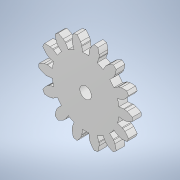
# Autodesk Inventor part: ｍ2歯数14ギアd3.99
Saved by Autodesk Inventor 2020.2 (Build 242310000, 310)
## iProperties
Created: 2020-03-09
Part Number: ｍ2歯数14ギアd3.99
Material: アルミニウム 2014-T4
Document SubType Name: Modeling
Designer: aoyam
Density: 2.8 g/cm^3
Appearance: サテン
Author: aoyam
Autodesk Inventor part; units mm, degrees
ref_plane "YZ Plane" through (0, 0, 0) normal (1, 0, 0) x (0, 1, 0)
ref_plane "XZ Plane" through (0, 0, 0) normal (0, 1, 0) x (-1, 0, 0)
ref_plane "XY Plane" through (0, 0, 0) normal (0, 0, 1) x (1, 0, 0)
sketch "スケッチ1" plane through (0, 0, 0) normal (0, 0, 1) x (1, 0, 0)
  arc A0 (3.0273, 14.808) -> (2.9636, 14.5404) centre (4.4576, 14.3261) ccw
  arc A1 (3.4088, 15.6481) -> (3.0273, 14.808) centre (7.0051, 13.5085) ccw
  arc A2 (4.6135, 17.1768) -> (3.4088, 15.6481) centre (9.7453, 11.8935) ccw
  arc A3 (0.4077, 14.5404) -> (0.344, 14.808) centre (-1.0864, 14.3261) ccw
  arc A4 (0.344, 14.808) -> (-0.0375, 15.6481) centre (-3.6338, 13.5085) ccw
  arc A5 (-0.0375, 15.6481) -> (-1.2422, 17.1768) centre (-6.374, 11.8935) ccw
  arc A6 (2.8028, 12.8925) -> (0.5685, 12.8925) centre (1.6856, 1.4469) ccw
  arc A7 (-1.2422, 17.1768) -> (-2.5014, 16.8894) centre (1.6856, 1.4469) ccw
  line L0 (2.8028, 12.8925) -> (2.9636, 14.5404)
  line L1 (0.5685, 12.8925) -> (0.4077, 14.5404)
  arc A8 (-6.0285, 13.4941) -> (-7.7772, 14.3487) centre (-10.1084, 7.362) ccw
  arc A9 (-7.7772, 14.3487) -> (-8.787, 13.5434) centre (1.6856, 1.4469) ccw
  arc A10 (-5.3203, 12.9027) -> (-6.0285, 13.4941) centre (-8.3404, 10.006) ccw
  arc A11 (-5.1468, 12.6893) -> (-5.3203, 12.9027) centre (-6.3999, 11.8479) ccw
  line L2 (-4.2869, 11.2744) -> (-5.1468, 12.6893)
  arc A12 (-2.9027, 14.067) -> (-2.844, 13.7982) centre (-1.405, 14.2534) ccw
  arc A13 (-2.9235, 14.9894) -> (-2.9027, 14.067) centre (1.2449, 14.6221) ccw
  arc A14 (-2.5014, 16.8894) -> (-2.9235, 14.9894) centre (4.4145, 14.3559) ccw
  line L3 (-2.2739, 12.2438) -> (-2.844, 13.7982)
  arc A15 (-2.2739, 12.2438) -> (-4.2869, 11.2744) centre (1.6856, 1.4469) ccw
  arc A16 (-10.4917, 8.954) -> (-12.4379, 8.9653) centre (-11.5069, 1.659) ccw
  arc A17 (-12.4379, 8.9653) -> (-12.9983, 7.8016) centre (1.6856, 1.4469) ccw
  arc A18 (-9.597, 8.7285) -> (-10.4917, 8.954) centre (-11.0611, 4.8083) ccw
  arc A19 (-9.3481, 8.6114) -> (-9.597, 8.7285) centre (-10.112, 7.3097) ccw
  line L4 (-7.9594, 7.7097) -> (-9.3481, 8.6114)
  arc A20 (-7.9239, 10.8264) -> (-7.7545, 10.6097) centre (-6.6554, 11.6442) ccw
  arc A21 (-8.343, 11.6485) -> (-7.9239, 10.8264) centre (-4.4279, 13.1261) ccw
  arc A22 (-8.787, 13.5434) -> (-8.343, 11.6485) centre (-1.4567, 14.2615) ccw
  line L5 (-6.5664, 9.4566) -> (-7.7545, 10.6097)
  arc A23 (-6.5664, 9.4566) -> (-7.9594, 7.7097) centre (1.6856, 1.4469) ccw
  arc A24 (-12.543, 2.927) -> (-14.3013, 2.0927) centre (-10.2925, -4.086) ccw
  arc A25 (-14.3013, 2.0927) -> (-14.3013, 0.8011) centre (1.6856, 1.4469) ccw
  arc A26 (-11.639, 3.112) -> (-12.543, 2.927) centre (-11.2573, -1.0552) ccw
  arc A27 (-11.3639, 3.1146) -> (-11.639, 3.112) centre (-11.4875, 1.6103) ccw
  line L6 (-9.7216, 2.9047) -> (-11.3639, 3.1146)
  arc A28 (-11.0419, 5.7281) -> (-10.7952, 5.6064) centre (-10.2538, 7.0153) ccw
  arc A29 (-11.7761, 6.2869) -> (-11.0419, 5.7281) centre (-8.8899, 9.317) ccw
  arc A30 (-12.9983, 7.8016) -> (-11.7761, 6.2869) centre (-6.7056, 11.6291) ccw
  line L7 (-9.2244, 5.0829) -> (-10.7952, 5.6064)
  arc A31 (-9.2244, 5.0829) -> (-9.7216, 2.9047) centre (1.6856, 1.4469) ccw
  arc A32 (-11.7761, -3.3931) -> (-12.9983, -4.9077) centre (-6.7056, -8.7352) ccw
  arc A33 (-12.9983, -4.9077) -> (-12.4379, -6.0714) centre (1.6856, 1.4469) ccw
  arc A34 (-11.0419, -2.8342) -> (-11.7761, -3.3931) centre (-8.8899, -6.4231) ccw
  arc A35 (-10.7952, -2.7126) -> (-11.0419, -2.8342) centre (-10.2538, -4.1214) ccw
  line L8 (-9.2244, -2.1891) -> (-10.7952, -2.7126)
  arc A36 (-11.639, -0.2182) -> (-11.3639, -0.2207) centre (-11.4875, 1.2835) ccw
  arc A37 (-12.543, -0.0332) -> (-11.639, -0.2182) centre (-11.2573, 3.949) ccw
  arc A38 (-14.3013, 0.8011) -> (-12.543, -0.0332) centre (-10.2925, 6.9799) ccw
  line L9 (-9.7216, -0.0108) -> (-11.3639, -0.2207)
  arc A39 (-9.7216, -0.0108) -> (-9.2244, -2.1891) centre (1.6856, 1.4469) ccw
  arc A40 (-8.343, -8.7546) -> (-8.787, -10.6495) centre (-1.4567, -11.3677) ccw
  arc A41 (-8.787, -10.6495) -> (-7.7772, -11.4548) centre (1.6856, 1.4469) ccw
  arc A42 (-7.9239, -7.9325) -> (-8.343, -8.7546) centre (-4.4279, -10.2323) ccw
  arc A43 (-7.7545, -7.7159) -> (-7.9239, -7.9325) centre (-6.6554, -8.7503) ccw
  line L10 (-6.5664, -6.5627) -> (-7.7545, -7.7159)
  arc A44 (-9.597, -5.8346) -> (-9.3481, -5.7176) centre (-10.112, -4.4159) ccw
  arc A45 (-10.4917, -6.0602) -> (-9.597, -5.8346) centre (-11.0611, -1.9145) ccw
  arc A46 (-12.4379, -6.0714) -> (-10.4917, -6.0602) centre (-11.5069, 1.2349) ccw
  line L11 (-7.9594, -4.8159) -> (-9.3481, -5.7176)
  arc A47 (-7.9594, -4.8159) -> (-6.5664, -6.5627) centre (1.6856, 1.4469) ccw
  arc A48 (-2.9235, -12.0956) -> (-2.5014, -13.9955) centre (4.4145, -11.4621) ccw
  arc A49 (-2.5014, -13.9955) -> (-1.2422, -14.2829) centre (1.6856, 1.4469) ccw
  arc A50 (-2.9027, -11.1731) -> (-2.9235, -12.0956) centre (1.2449, -11.7282) ccw
  arc A51 (-2.844, -10.9044) -> (-2.9027, -11.1731) centre (-1.405, -11.3595) ccw
  line L12 (-2.2739, -9.3499) -> (-2.844, -10.9044)
  arc A52 (-5.3203, -10.0088) -> (-5.1468, -9.7954) centre (-6.3999, -8.9541) ccw
  arc A53 (-6.0285, -10.6003) -> (-5.3203, -10.0088) centre (-8.3404, -7.1122) ccw
  arc A54 (-7.7772, -11.4548) -> (-6.0285, -10.6003) centre (-10.1084, -4.4682) ccw
  line L13 (-4.2869, -8.3805) -> (-5.1468, -9.7954)
  arc A55 (-4.2869, -8.3805) -> (-2.2739, -9.3499) centre (1.6856, 1.4469) ccw
  arc A56 (3.4088, -12.7543) -> (4.6135, -14.2829) centre (9.7453, -8.9997) ccw
  arc A57 (4.6135, -14.2829) -> (5.8727, -13.9955) centre (1.6856, 1.4469) ccw
  arc A58 (3.0273, -11.9141) -> (3.4088, -12.7543) centre (7.0051, -10.6147) ccw
  arc A59 (2.9636, -11.6465) -> (3.0273, -11.9141) centre (4.4576, -11.4323) ccw
  line L14 (2.8028, -9.9987) -> (2.9636, -11.6465)
  arc A60 (0.344, -11.9141) -> (0.4077, -11.6465) centre (-1.0864, -11.4323) ccw
  arc A61 (-0.0375, -12.7543) -> (0.344, -11.9141) centre (-3.6338, -10.6147) ccw
  arc A62 (-1.2422, -14.2829) -> (-0.0375, -12.7543) centre (-6.374, -8.9997) ccw
  line L15 (0.5685, -9.9987) -> (0.4077, -11.6465)
  arc A63 (0.5685, -9.9987) -> (2.8028, -9.9987) centre (1.6856, 1.4469) ccw
  arc A64 (9.3998, -10.6003) -> (11.1484, -11.4548) centre (13.4797, -4.4682) ccw
  arc A65 (11.1484, -11.4548) -> (12.1583, -10.6495) centre (1.6856, 1.4469) ccw
  arc A66 (8.6916, -10.0088) -> (9.3998, -10.6003) centre (11.7116, -7.1122) ccw
  arc A67 (8.5181, -9.7954) -> (8.6916, -10.0088) centre (9.7712, -8.9541) ccw
  line L16 (7.6582, -8.3805) -> (8.5181, -9.7954)
  arc A68 (6.274, -11.1731) -> (6.2153, -10.9044) centre (4.7762, -11.3595) ccw
  arc A69 (6.2948, -12.0956) -> (6.274, -11.1731) centre (2.1263, -11.7282) ccw
  arc A70 (5.8727, -13.9955) -> (6.2948, -12.0956) centre (-1.0432, -11.4621) ccw
  line L17 (5.6452, -9.3499) -> (6.2153, -10.9044)
  arc A71 (5.6452, -9.3499) -> (7.6582, -8.3805) centre (1.6856, 1.4469) ccw
  arc A72 (13.863, -6.0602) -> (15.8092, -6.0714) centre (14.8782, 1.2349) ccw
  arc A73 (15.8092, -6.0714) -> (16.3696, -4.9077) centre (1.6856, 1.4469) ccw
  arc A74 (12.9683, -5.8346) -> (13.863, -6.0602) centre (14.4324, -1.9145) ccw
  arc A75 (12.7193, -5.7176) -> (12.9683, -5.8346) centre (13.4833, -4.4159) ccw
  line L18 (11.3307, -4.8159) -> (12.7193, -5.7176)
  arc A76 (11.2952, -7.9325) -> (11.1257, -7.7159) centre (10.0267, -8.7503) ccw
  arc A77 (11.7142, -8.7546) -> (11.2952, -7.9325) centre (7.7992, -10.2323) ccw
  arc A78 (12.1583, -10.6495) -> (11.7142, -8.7546) centre (4.828, -11.3677) ccw
  line L19 (9.9377, -6.5627) -> (11.1257, -7.7159)
  arc A79 (9.9377, -6.5627) -> (11.3307, -4.8159) centre (1.6856, 1.4469) ccw
  arc A80 (15.9142, -0.0332) -> (17.6726, 0.8011) centre (13.6637, 6.9799) ccw
  arc A81 (17.6726, 0.8011) -> (17.6726, 2.0927) centre (1.6856, 1.4469) ccw
  arc A82 (15.0103, -0.2182) -> (15.9142, -0.0332) centre (14.6285, 3.949) ccw
  arc A83 (14.7352, -0.2207) -> (15.0103, -0.2182) centre (14.8587, 1.2835) ccw
  line L20 (13.0929, -0.0108) -> (14.7352, -0.2207)
  arc A84 (14.4132, -2.8342) -> (14.1665, -2.7126) centre (13.6251, -4.1214) ccw
  arc A85 (15.1474, -3.3931) -> (14.4132, -2.8342) centre (12.2612, -6.4231) ccw
  arc A86 (16.3696, -4.9077) -> (15.1474, -3.3931) centre (10.0769, -8.7352) ccw
  line L21 (12.5957, -2.1891) -> (14.1665, -2.7126)
  arc A87 (12.5957, -2.1891) -> (13.0929, -0.0108) centre (1.6856, 1.4469) ccw
  arc A88 (15.1474, 6.2869) -> (16.3696, 7.8016) centre (10.0769, 11.6291) ccw
  arc A89 (16.3696, 7.8016) -> (15.8092, 8.9653) centre (1.6856, 1.4469) ccw
  arc A90 (14.4132, 5.7281) -> (15.1474, 6.2869) centre (12.2612, 9.317) ccw
  arc A91 (14.1665, 5.6064) -> (14.4132, 5.7281) centre (13.6251, 7.0153) ccw
  line L22 (12.5957, 5.0829) -> (14.1665, 5.6064)
  arc A92 (15.0103, 3.112) -> (14.7352, 3.1146) centre (14.8587, 1.6103) ccw
  arc A93 (15.9142, 2.927) -> (15.0103, 3.112) centre (14.6285, -1.0552) ccw
  arc A94 (17.6726, 2.0927) -> (15.9142, 2.927) centre (13.6637, -4.086) ccw
  line L23 (13.0929, 2.9047) -> (14.7352, 3.1146)
  arc A95 (13.0929, 2.9047) -> (12.5957, 5.0829) centre (1.6856, 1.4469) ccw
  arc A96 (11.7142, 11.6485) -> (12.1583, 13.5434) centre (4.828, 14.2615) ccw
  arc A97 (12.1583, 13.5434) -> (11.1484, 14.3487) centre (1.6856, 1.4469) ccw
  arc A98 (11.2952, 10.8264) -> (11.7142, 11.6485) centre (7.7992, 13.1261) ccw
  arc A99 (11.1257, 10.6097) -> (11.2952, 10.8264) centre (10.0267, 11.6442) ccw
  line L24 (9.9377, 9.4566) -> (11.1257, 10.6097)
  arc A100 (12.9683, 8.7285) -> (12.7193, 8.6114) centre (13.4833, 7.3097) ccw
  arc A101 (13.863, 8.954) -> (12.9683, 8.7285) centre (14.4324, 4.8083) ccw
  arc A102 (15.8092, 8.9653) -> (13.863, 8.954) centre (14.8782, 1.659) ccw
  line L25 (11.3307, 7.7097) -> (12.7193, 8.6114)
  arc A103 (11.3307, 7.7097) -> (9.9377, 9.4566) centre (1.6856, 1.4469) ccw
  arc A104 (6.2948, 14.9894) -> (5.8727, 16.8894) centre (-1.0432, 14.3559) ccw
  arc A105 (5.8727, 16.8894) -> (4.6135, 17.1768) centre (1.6856, 1.4469) ccw
  arc A106 (6.274, 14.067) -> (6.2948, 14.9894) centre (2.1263, 14.6221) ccw
  arc A107 (6.2153, 13.7982) -> (6.274, 14.067) centre (4.7762, 14.2534) ccw
  line L26 (5.6452, 12.2438) -> (6.2153, 13.7982)
  arc A108 (8.6916, 12.9027) -> (8.5181, 12.6893) centre (9.7712, 11.8479) ccw
  arc A109 (9.3998, 13.4941) -> (8.6916, 12.9027) centre (11.7116, 10.006) ccw
  arc A110 (11.1484, 14.3487) -> (9.3998, 13.4941) centre (13.4797, 7.362) ccw
  line L27 (7.6582, 11.2744) -> (8.5181, 12.6893)
  arc A111 (7.6582, 11.2744) -> (5.6452, 12.2438) centre (1.6856, 1.4469) ccw
  circle A112 centre (1.6856, 1.4469) radius 1.995
  circle A113 centre (1.6856, 1.4469) radius 11.5
  point P0 (0, 0)
  point P1 (6.2153, 13.7982)
  point P2 (6.274, 14.067)
  point P3 (6.2948, 14.9894)
  point P4 (5.8727, 16.8894)
  point P5 (4.6135, 17.1768)
  point P6 (3.4088, 15.6481)
  point P7 (3.0273, 14.808)
  point P8 (0.344, 14.808)
  point P9 (-0.0375, 15.6481)
  point P10 (-1.2422, 17.1768)
  point P11 (-2.5014, 16.8894)
  point P12 (-2.9235, 14.9894)
  point P13 (-2.9027, 14.067)
  point P14 (-2.844, 13.7982)
  point P15 (-2.2739, 12.2438)
  point P16 (-4.2869, 11.2744)
  point P17 (-5.1468, 12.6893)
  point P18 (-5.3203, 12.9027)
  point P19 (-6.0285, 13.4941)
  point P20 (-7.7772, 14.3487)
  point P21 (-8.787, 13.5434)
  point P22 (-8.343, 11.6485)
  point P23 (-7.7545, 10.6097)
  point P24 (-6.5664, 9.4566)
  point P25 (-7.9594, 7.7097)
  point P26 (-9.3481, 8.6114)
  point P27 (-9.597, 8.7285)
  point P28 (-10.4917, 8.954)
  point P29 (-12.4379, 8.9653)
  point P30 (-12.9983, 7.8016)
  point P31 (-11.7761, 6.2869)
  point P32 (-11.0419, 5.7281)
  point P33 (-10.7952, 5.6064)
  point P34 (-11.3639, 3.1146)
  point P35 (-11.639, 3.112)
  point P36 (-12.543, 2.927)
  point P37 (-14.3013, 2.0927)
  point P38 (-14.3013, 0.8011)
  point P39 (-12.543, -0.0332)
  point P40 (-11.639, -0.2182)
  point P41 (-11.3639, -0.2207)
  point P42 (-9.7216, -0.0108)
  point P43 (-10.7952, -2.7126)
  point P44 (-11.0419, -2.8342)
  point P45 (-11.7761, -3.3931)
  point P46 (-12.9983, -4.9077)
  point P47 (-12.4379, -6.0714)
  point P48 (-10.4917, -6.0602)
  point P49 (-9.597, -5.8346)
  point P50 (-9.3481, -5.7176)
  point P51 (-7.9239, -7.9325)
  point P52 (-8.343, -8.7546)
  point P53 (-8.787, -10.6495)
  point P54 (-7.7772, -11.4548)
  point P55 (-6.0285, -10.6003)
  point P56 (-5.3203, -10.0088)
  point P57 (-5.1468, -9.7954)
  point P58 (-4.2869, -8.3805)
  point P59 (-2.844, -10.9044)
  point P60 (-2.9027, -11.1731)
  point P61 (-2.9235, -12.0956)
  point P62 (-2.5014, -13.9955)
  point P63 (-1.2422, -14.2829)
  point P64 (-0.0375, -12.7543)
  point P65 (0.344, -11.9141)
  point P66 (0.5685, -9.9987)
  point P67 (2.8028, -9.9987)
  point P68 (3.0273, -11.9141)
  point P69 (3.4088, -12.7543)
  point P70 (4.6135, -14.2829)
  point P71 (5.8727, -13.9955)
  point P72 (6.2948, -12.0956)
  point P73 (6.274, -11.1731)
  point P74 (5.6452, -9.3499)
  point P75 (7.6582, -8.3805)
  point P76 (8.6916, -10.0088)
  point P77 (9.3998, -10.6003)
  point P78 (11.1484, -11.4548)
  point P79 (12.1583, -10.6495)
  point P80 (11.2952, -7.9325)
  point P81 (11.1257, -7.7159)
  point P82 (12.7193, -5.7176)
  point P83 (12.9683, -5.8346)
  point P84 (13.863, -6.0602)
  point P85 (15.8092, -6.0714)
  point P86 (16.3696, -4.9077)
  point P87 (15.1474, -3.3931)
  point P88 (14.4132, -2.8342)
  point P89 (14.1665, -2.7126)
  point P90 (14.7352, -0.2207)
  point P91 (15.0103, -0.2182)
  point P92 (15.9142, -0.0332)
  point P93 (17.6726, 0.8011)
  point P94 (17.6726, 2.0927)
  point P95 (15.9142, 2.927)
  point P96 (15.0103, 3.112)
  point P97 (13.0929, 2.9047)
  point P98 (12.5957, 5.0829)
  point P99 (14.4132, 5.7281)
  point P100 (15.1474, 6.2869)
  point P101 (16.3696, 7.8016)
  point P102 (15.8092, 8.9653)
  point P103 (13.863, 8.954)
  point P104 (12.9683, 8.7285)
  point P105 (11.3307, 7.7097)
  point P106 (9.9377, 9.4566)
  point P107 (11.2952, 10.8264)
  point P108 (11.7142, 11.6485)
  point P109 (12.1583, 13.5434)
  point P110 (11.1484, 14.3487)
  point P111 (9.3998, 13.4941)
  point P112 (8.5181, 12.6893)
  dimension "d2" = 360
  dimension "d4" = 3.99
  constraints: 224 point on circle, 114 centre point, 56 end point, 3 coincident, 568 other
  measures "d4" diameter of A112
extrude "押し出し1" add sketch "スケッチ1" along normal blind 3
